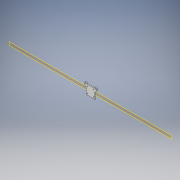
# Autodesk Inventor part: CarriagePlate
Saved by Autodesk Inventor 2019 (Build 230136000, 136)
## iProperties
Created: 2019-05-07
Part Number: CarriagePlate
Material: Generic
Document SubType Name: Modeling
Designer: Alex Jones
Density: 1 g/cm^3
Appearance: Default
Author: Alex Jones
Autodesk Inventor part; units mm, degrees
ref_plane "YZ Plane" through (0, 0, 0) normal (1, 0, 0) x (0, 1, 0)
ref_plane "XZ Plane" through (0, 0, 0) normal (0, 1, 0) x (-1, 0, 0)
ref_plane "XY Plane" through (0, 0, 0) normal (0, 0, 1) x (1, 0, 0)
ref_plane "Work Plane1" through (0, 0, 0) normal (0, 0, 1) x (1, 0, 0)
sketch "Sketch1" plane through (0, 0, 0) normal (0, 0, 1) x (1, 0, 0)
  circle A0 centre (-473.5705, 17.8) radius 2.5 projected
  circle A1 centre (-473.5705, 17.8) radius 9.9 construction
  circle A2 centre (-473.5705, -25) radius 2.5 projected
  circle A3 centre (-473.5705, -25) radius 9.9 construction
  line L0 (-473.5705, -25) -> (-473.5705, 17.8) construction
  circle A4 centre (-513.5705, 17.8) radius 2.5 projected
  circle A5 centre (-513.5705, 17.8) radius 9.9 construction
  circle A6 centre (-513.5705, -25) radius 2.5 projected
  circle A7 centre (-513.5705, -25) radius 9.9 construction
  line L1 (-513.5705, 17.8) -> (-513.5705, -25) construction
  line L2 (-513.5705, 17.8) -> (-473.5705, 17.8) construction
  line L3 (-513.5705, -25) -> (-473.5705, -25) construction
  line L4 (-463.6705, 18.91) -> (-463.6705, -34.9)
  line L5 (-463.6705, -34.9) -> (-523.4705, -34.9)
  line L6 (-523.4705, -34.9) -> (-523.4705, 18.91)
  line L7 (-519.0445, 27.8) -> (-468.0964, 27.8)
  line L8 (-463.6705, 27.8) -> (-453.6705, 27.8) construction
  line L9 (-452.9305, 18.91) -> (-463.6705, 18.91)
  line L10 (-534.2105, 28.86) -> (-534.2105, 18.91)
  line L11 (-534.2105, 18.91) -> (-523.4705, 18.91)
  circle A8 centre (-460.5505, 28.86) radius 2.75
  line L12 (-473.5705, -3.6) -> (-408.7211, -3.6) construction
  line L13 (-564.232, 28.86) -> (-376.8573, 28.86) construction
  arc A9 (-452.9305, 28.86) -> (-468.0964, 27.8) centre (-460.5505, 28.86) ccw
  line L14 (-493.5705, 27.8) -> (-493.5705, -34.9) construction
  line L15 (-452.9305, 28.86) -> (-452.9305, 18.91)
  circle A10 centre (-526.5905, 28.86) radius 2.75
  arc A11 (-519.0445, 27.8) -> (-534.2105, 28.86) centre (-526.5905, 28.86) ccw
  point P0 (0, 0)
  point P1 (-514.2552, 27.8)
  point P2 (-534.2105, 10.8915)
  dimension "d2" = 10
  dimension "d14" = 0
  dimension "d16" = 32.46
  dimension "d17" = 33.02
  dimension "d18" = 5.5
  dimension "d19" = 7.62
  dimension "d20" = 8.89
  constraints: 32 end point, 5 perpendicular, 4 centre point, 4 point on circle, 4 symmetric about line, 4 tangent, 3 horizontal, 3 midpoint, 3 point on line, 2 coincident, 1 parallel, 1 vertical, 2 other
  measures "d2" distance between parallel lines of L2 L7
  measures "d14" distance from line of L13 A8.centre
  measures "d16" distance from line of L12 A8.centre
  measures "d17" distance from line of L14 A8.centre
  measures "d18" diameter of A10
  measures "d19" radius of A11
  measures "d20" distance between parallel lines of L7 L9
extrude "Extrusion1" add sketch "Sketch1" along normal blind 6.35
sketch "Sketch2" plane through (0, 0, 6.35) normal (0, 0, 1) x (1, 0, 0)
  line L0 (-463.6705, 18.91) -> (-452.9305, 18.91) projected
  line L1 (-452.9305, 18.91) -> (-463.6705, 8.17)
  line L2 (-534.2105, 28.86) -> (-534.2105, 18.91) projected
  line L3 (-534.2105, 18.91) -> (-523.4705, 8.17)
  line L4 (-523.4705, 18.91) -> (-523.4705, -34.9) projected
  line L5 (-534.2105, 18.91) -> (-523.4705, 18.91) projected
  line L6 (-534.2105, 18.91) -> (-523.4705, 18.91)
  line L7 (-523.4705, 8.17) -> (-523.4705, 18.91)
  line L8 (-463.6705, -34.9) -> (-463.6705, 18.91) projected
  line L9 (-463.6705, 8.17) -> (-463.6705, 18.91)
  line L10 (-452.9305, 18.91) -> (-463.6705, 18.91)
  point P0 (0, 0)
  point P1 (-548.4705, 27.8)
  point P2 (-548.4705, 15.264)
  dimension "d6" = 45
  constraints: 12 end point, 3 perpendicular, 3 point on line, 1 vertical, 1 other
  measures "d6" angle of L5 L3
extrude "Extrusion2" add sketch "Sketch2" against normal up to surface (6.35 mm away)
body "Solid1"
